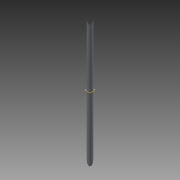
# Autodesk Inventor part: guida_Z
Saved by Autodesk Inventor 2014 SP1 (Build 180222100, 222)
## iProperties
Created: 2015-04-08
Part Number: guida_Z
Material: Generic
Document SubType Name: Modeling
Designer: Giorgio Nuzzo
Density: 1 g/cm^3
Appearance: Default
d0: 300,000 mm
d1: 0,00 deg
Author: Giorgio Nuzzo
Autodesk Inventor part; units mm, degrees
ref_plane "YZ Plane" through (0, 0, 0) normal (1, 0, 0) x (0, 1, 0)
ref_plane "XZ Plane" through (0, 0, 0) normal (0, 1, 0) x (-1, 0, 0)
ref_plane "XY Plane" through (0, 0, 0) normal (0, 0, 1) x (1, 0, 0)
ref_plane "Work Plane1" through (-6.5765, 0, 5) normal (0, 0, 1) x (1, 0, 0)
sketch "Sketch1" plane through (-6.5765, 0, 5) normal (0, 0, 1) x (1, 0, 0)
  circle A0 centre (0, 0) radius 5 projected
  point P0 (6.5765, 0)
extrude "Extrusion1" add sketch "Sketch1" against normal blind 300
ref_plane "Work Plane2" through (-6.5765, 0, -145) normal (0, 0, -1) x (-1, 0, 0)
body "Solid1"
